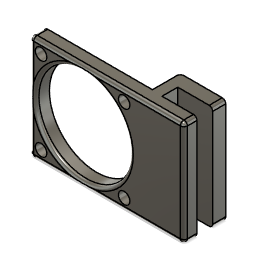
bracketAirFan (Autodesk Fusion 360 design; units mm, degrees)
Autodesk Fusion 360 part; units mm, degrees
sketch "Schizzo1" plane through (0, 0, 0) normal (0, 0, 1) x (1, 0, 0)
  line L0 (50, 60) -> (73.8, 60)
  line L1 (73.8, 60) -> (73.8, 36.2)
  line L2 (73.8, 36.2) -> (50, 36.2)
  line L3 (50, 36.2) -> (50, 60)
  circle A0 centre (61.9, 48.1) radius 13.5
  circle A1 centre (50, 60) radius 1.65
  circle A2 centre (73.8, 60) radius 1.65
  circle A3 centre (73.8, 36.2) radius 1.65
  circle A4 centre (50, 36.2) radius 1.65
  line L4 (76.9, 63.1) -> (46.9, 63.1)
  line L5 (46.9, 63.1) -> (46.9, 33.1)
  line L6 (46.9, 33.1) -> (76.9, 33.1)
  line L7 (76.9, 33.1) -> (76.9, 63.1)
  line L8 (76.9, 63.1) -> (46.9, 33.1) construction
  line L9 (46.9, 63.1) -> (76.9, 33.1) construction
  point P0 (61.9, 48.1)
  dimension "d1" = 23.8
  dimension "d2" = 23.8
  dimension "d3" = 27
  dimension "d4" = 3.3
  dimension "d5" = 3.3
  dimension "d6" = 3.3
  dimension "d7" = 3.3
  dimension "d8" = 30
  dimension "d9" = 30
  constraint horizontal L0
  constraint vertical L1
  constraint horizontal L2
  constraint vertical L3
  constraint coincident L0.start L3.end
  constraint coincident L0.end L1.start
  constraint coincident L1.end L2.start
  constraint coincident L2.end L3.start
  constraint horizontal L4
  constraint perpendicular L4 L5
  constraint parallel L4 L6
  constraint parallel L5 L7
  constraint coincident L8 P0
  constraint coincident L9 P0
  constraint coincident P0 A0.centre
  measures "d1" distance of L0.start L0.end
  measures "d2" distance of L0.start L2.end
  measures "d3" diameter of A0
  measures "d4" diameter of A1
  measures "d5" diameter of A2
  measures "d6" diameter of A3
  measures "d7" diameter of A4
  measures "d8" distance of L5.end L6.end
  measures "d9" distance of L4.end L5.end
extrude "Estrusione1" add sketch "Schizzo1" along normal blind 4 contours L0 L3 A0 A1 | L0 L1 A0 A2 | L2 L3 A0 A4 | L1 L2 A0 A3 | L4 L5 L6 L7
extrude "Estrusione2" add 1 faces at (76.9, 43.1, 1.3333) along direction (1, 0, 0) blind 3
box "PrimitivaParallelepipedo1" add length 30 width 3 height 8 placed x (0, 1, 0) y (1, 0, 0) z (0, 0, -1) at (76.9, 33.1, 0)
extrude "Estrusione3" cut 1 faces at (76.9, 53.1, -2.6667) along direction (1, 0, 0) blind 1
extrude "Estrusione4" add 1 faces at (79.9, 43.1, 0) along direction (1, 0, 0) blind 1
sketch "Schizzo3" plane through (80.9, 0, 0) normal (1, 0, 0) x (0, 0, -1)
  line L0 (8, 63.1) -> (-4, 63.1)
  line L1 (-4, 63.1) -> (-4, 33.1)
  line L2 (-4, 33.1) -> (8, 33.1)
  line L3 (8, 33.1) -> (8, 63.1)
  line L4 (2, 63.1) -> (-0.25, 63.1)
  line L5 (2, 63.1) -> (4.25, 63.1)
  line L6 (-0.25, 63.1) -> (4.25, 63.1)
  line L7 (4.25, 63.1) -> (4.25, 33.1)
  line L8 (4.25, 33.1) -> (-0.25, 33.1)
  line L9 (-0.25, 33.1) -> (-0.25, 63.1)
  dimension "d23" = 2.25
  dimension "d24" = 2.25
  constraint midpoint L0 L4.start
  constraint perpendicular L1 L4
  constraint parallel L0 L5
  constraint horizontal L6
  constraint vertical L7
  constraint horizontal L8
  constraint vertical L9
  constraint coincident L2 L7.end
  measures "d23" distance of L4.start L4.end
  measures "d24" distance of L4.start L5.end
extrude "Estrusione5" add sketch "Schizzo3" along normal blind 10 contours L0 L2 L3 L7 | L0 L1 L2 L9
fillet "Raccordo1" radius 1 4 edges at (90.9, 63.1, 2.125) (90.9, 33.1, 2.125) (90.9, 33.1, -6.125) (90.9, 63.1, -6.125)
fillet "Raccordo2" radius 1 2 edges at (46.9, 63.1, 2) (46.9, 33.1, 2)
fillet "Raccordo3" radius 1 8 edges at (90.9, 48.1, 4) (90.6071, 33.3929, 4) (68.9, 33.1, 4) (47.1929, 33.3929, 4) (46.9, 48.1, 4) (47.1929, 62.8071, 4) (68.9, 63.1, 4) (90.6071, 62.8071, 4)
fillet "Raccordo4" radius 1 1 edges at (49.3136, 52.9818, 4)
fillet "Raccordo5" radius 1 1 edges at (77.9, 48.1, -8)
